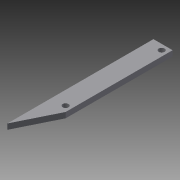
# Autodesk Inventor part: Spacer
Saved by Autodesk Inventor 2013 (Build 170138000, 138)
## iProperties
Created: 2013-02-01
Part Number: Spacer
Material: Generic
Document SubType Name: Modeling
Designer: actoennies
Density: 1 g/cm^3
Author: actoennies
Autodesk Inventor part; units mm, degrees
ref_plane "YZ Plane" through (0, 0, 0) normal (1, 0, 0) x (0, 1, 0)
ref_plane "XZ Plane" through (0, 0, 0) normal (0, 1, 0) x (-1, 0, 0)
ref_plane "XY Plane" through (0, 0, 0) normal (0, 0, 1) x (1, 0, 0)
sketch "Sketch1" plane through (0, 0, 0) normal (0, 1, 0) x (-1, 0, 0)
  circle A0 centre (130.175, -139.7) radius 3.3782
  circle A1 centre (130.175, -28.4093) radius 3.3782
  line L0 (146.05, 23.2231) -> (123.825, -22.0593)
  line L1 (123.825, -22.0593) -> (123.825, -146.05)
  line L2 (123.825, -146.05) -> (146.05, -146.05)
  line L3 (146.05, -146.05) -> (146.05, 23.2231)
  point P0 (0, 0)
  point P1 (0, 0)
  dimension "d0" = 22.225
  constraints: 8 end point, 2 centre point, 2 vertical, 10 other
  measures "d0" distance of L1.end L2.end
extrude "Extrusion1" add sketch "Sketch1" along normal blind 6.35
body "Solid1"
